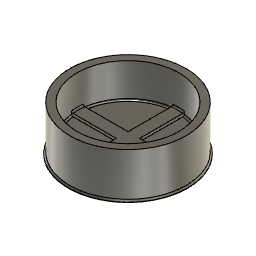
Tappo cucina v3 (Autodesk Fusion 360 design; units mm, degrees)
Autodesk Fusion 360 part; units mm, degrees
sketch "Schizzo5" plane through (0, 0, 0) normal (0, 0, 1) x (1, 0, 0)
  circle A0 centre (0, 0) radius 20.25
  dimension "d11" = 40.5
  constraint coincident A0.centre origin
  measures "d11" diameter of A0
extrude "Estrusione3" add sketch "Schizzo5" along normal blind 0.2
sketch "Schizzo6" plane through (0, 0, 0.2) normal (0, 0, 1) x (-1, 0, 0)
  circle A0 centre (0, 0) radius 20.25
  circle A1 centre (0, 0) radius 20
  dimension "d14" = 40
  constraint coincident A0.centre A1.centre
  measures "d14" diameter of A1
extrude "Estrusione4" add sketch "Schizzo6" along normal blind 3 contours A1
sketch "Schizzo7" plane through (0, 0, 3.2) normal (0, 0, 1) x (-1, 0, 0)
  circle A0 centre (0, 0) radius 20
  circle A1 centre (0, 0) radius 18.5
  dimension "d17" = 37
  constraint coincident A0.centre A1.centre
  measures "d17" diameter of A1
extrude "Estrusione5" add sketch "Schizzo7" along normal blind 11.8
sketch "Schizzo8" plane through (0, 0, 3.2) normal (0, 0, 1) x (-1, 0, 0)
  circle A0 centre (0, 0) radius 18.5
  circle A1 centre (0, 0) radius 17.5
  dimension "d20" = 35
  constraint coincident A0.centre A1.centre
  measures "d20" diameter of A1
extrude "Estrusione6" add sketch "Schizzo8" along normal blind 11.8
sketch "Schizzo9" plane through (0, 0, 0) normal (0, 1, 0) x (1, 0, 0)
extrude "Estrusione7" add 1 faces at (1.5731, -1.2545, 0) along direction (0, 0, -1) blind 0.4
sketch "Schizzo10" plane through (0, 0, 0) normal (0, 0, 1) x (1, 0, 0)
  circle A0 centre (0, 0) radius 20.4969
  circle A1 centre (0, 0) radius 20.2493
  constraint coincident A0.centre A1.centre
move_body "Sposta1" bodies 1 to x (1, 0, 0) y (0, 1, 0) z (0, 0, 1) at (0, 0, 0.4)
extrude "Estrusione8" add sketch "Schizzo10" along normal blind 0.6
chamfer "Smusso1" distance 0.4969 angle 45 1 edges at (-19.1098, -7.412, 0.6) measured on face at (-19.0549, 6.9433, 0.6)
sketch "Schizzo11" plane through (0, 0, 3.6) normal (0, 0, 1) x (-1, 0, 0)
  circle A0 centre (0, 0) radius 17.5
  line L0 (1.9934, -17.3861) -> (1.9934, 17.3861)
  line L1 (-1.9934, 17.3861) -> (-1.9934, -17.3861)
  line L2 (17.3847, -2.0054) -> (-17.3847, -2.0054)
  line L3 (-17.3847, 2.0054) -> (17.3847, 2.0054)
  constraint coincident A0 L0.start
  constraint coincident A0 L0.end
  constraint vertical L0
  constraint coincident A0 L1.start
  constraint coincident A0 L1.end
  constraint parallel L0 L1
  constraint coincident A0 L2.start
  constraint coincident A0 L2.end
  constraint horizontal L2
  constraint coincident A0 L3.start
  constraint coincident A0 L3.end
  constraint perpendicular L1 L3
extrude "Estrusione9" add sketch "Schizzo11" along normal blind 1 contours A0 L0 L2 L3 | A0 L0 L1 L3 | L0 L1 L2 L3 | A0 L0 L1 L2 | A0 L1 L2 L3
fillet "Raccordo2" radius 0.5 8 edges at (-12.3701, 12.3786, 3.6) (0, 17.5, 4.6) (12.3701, 12.3786, 3.6) (12.3701, -12.3786, 3.6) (0, -17.5, 4.6) (17.5, 0, 4.6) (-12.3701, -12.3786, 3.6) (-17.5, 0, 4.6)
